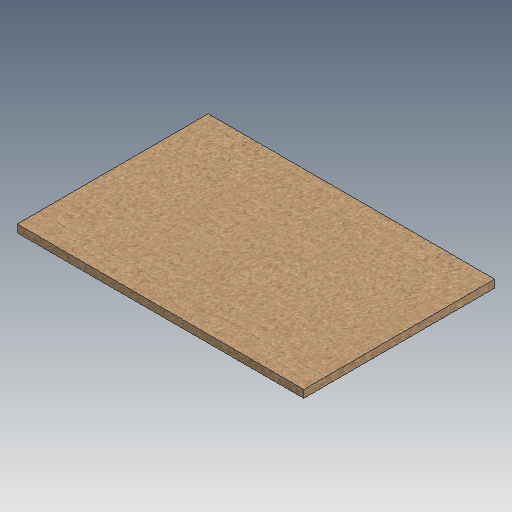
# Autodesk Inventor part: Placa de Mecanizado
Saved by Autodesk Inventor 2020.3 (Build 243373000, 373)
## iProperties
Created: 2020-06-06
Part Number: Placa de Mecanizado
Material: MDF Medium Density Fiberboard
Document SubType Name: Modeling
Designer: Pipi
Density: 0.8 g/cm^3
Appearance: Cardboard - Corrugated
Author: Pipi
Autodesk Inventor part; units mm, degrees
ref_plane "YZ Plane" through (0, 0, 0) normal (1, 0, 0) x (0, 1, 0)
ref_plane "XZ Plane" through (0, 0, 0) normal (0, 1, 0) x (-1, 0, 0)
ref_plane "XY Plane" through (0, 0, 0) normal (0, 0, 1) x (1, 0, 0)
sketch "Boceto1" plane through (0, 0, 0) normal (0, 1, 0) x (-1, 0, 0)
  line L0 (3.1255, 15.8014) -> (153.1255, 15.8014)
  line L1 (153.1255, 15.8014) -> (153.1255, -84.1986)
  line L2 (153.1255, -84.1986) -> (3.1255, -84.1986)
  line L3 (3.1255, -84.1986) -> (3.1255, 15.8014)
  point P0 (0, 0)
  dimension "d0" = 150
  dimension "d1" = 100
  constraints: 8 end point, 3 perpendicular, 1 horizontal
  measures "d0" distance of L0.start L0.end
  measures "d1" distance of L0.end L1.end
extrude "Extrusión1" add sketch "Boceto1" along normal blind 4
sketch "Boceto2" plane through (0, 4, 0) normal (0, 1, 0) x (1, 0, 0)
  point P0 (0, 0)
